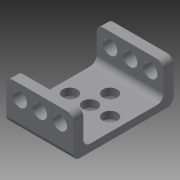
# Autodesk Inventor part: Pantilt
Saved by Autodesk Inventor 2014 (Build 180170000, 170)
## iProperties
Created: 2014-03-07
Part Number: Pantilt
Material: Générique
Document SubType Name: Modeling
Designer: Grégoire
Density: 1 g/cm^3
Appearance: Par défaut
Author: Grégoire
Autodesk Inventor part; units mm, degrees
ref_plane "YZ Plane" through (0, 0, 0) normal (1, 0, 0) x (0, 1, 0)
ref_plane "XZ Plane" through (0, 0, 0) normal (0, 1, 0) x (-1, 0, 0)
ref_plane "XY Plane" through (0, 0, 0) normal (0, 0, 1) x (1, 0, 0)
sketch "Esquisse5" plane through (0, 0, 0) normal (0, 0, 1) x (1, 0, 0)
  line L0 (0, 0) -> (20, 0)
  line L1 (20, 0) -> (20, 30)
  line L2 (20, 30) -> (0, 30)
  line L3 (0, 30) -> (0, 0)
  line L4 (10, 0) -> (10, 30) construction
  circle A0 centre (10, 9) radius 2.15
  circle A1 centre (10, 15) radius 2.15
  circle A2 centre (10, 21) radius 2.15
  line L5 (10, 15) -> (20, 15) construction
  circle A3 centre (16, 15) radius 2.15
  circle A4 centre (4, 15) radius 2.15
  circle A5 centre (10, 15) radius 2.15
  dimension "d61" = 20
  dimension "d62" = 30
  dimension "d64" = 4.3
  dimension "d67" = 6
  dimension "d74" = 6
  dimension "d77" = 6
  constraints: 12 end point, 6 centre point, 4 midpoint, 3 horizontal, 2 parallel, 2 perpendicular, 1 coincident, 1 point on line, 1 vertical, 10 other
  measures "d61" distance of L0.start L0.end
  measures "d62" distance of L2.end L0.start
  measures "d64" diameter of A0
  measures "d67" distance of A0.centre L5.start
  measures "d74" distance of L5.start A3.centre
  measures "d77" distance of L5.start A4.centre
extrude "Extrusion5" add sketch "Esquisse5" along normal blind 2.2
sketch "Esquisse9" plane through (0, 0, 2.2) normal (0, 0, 1) x (1, 0, 0)
  line L0 (20, 0) -> (20, 30) construction
  line L1 (0, 30) -> (0, 0) construction
  line L2 (0, 30) -> (20, 30)
  line L3 (20, 30) -> (20, 27)
  line L4 (20, 27) -> (0, 27)
  line L5 (0, 27) -> (0, 30)
  line L6 (0, 15) -> (20, 15) construction
  line L7 (20, 0) -> (0, 0) construction
  line L8 (0, 0) -> (20, 0)
  line L9 (20, 0) -> (20, 3)
  line L10 (20, 3) -> (0, 3)
  line L11 (0, 3) -> (0, 0)
  dimension "d102" = 3
  constraints: 20 end point, 4 symmetric about line, 2 midpoint, 2 parallel, 1 horizontal, 1 perpendicular, 1 point on line
  measures "d102" distance between parallel lines of L2 L4
extrude "Extrusion9" add sketch "Esquisse9" along normal blind 10
sketch "Esquisse10" plane through (0, 0, 0) normal (0, -1, 0) x (1, 0, 0)
  line L0 (0, 0) -> (20, 0) construction
  line L1 (20, 0) -> (20, 12.2) construction
  line L2 (0, 12.2) -> (20, 12.2) construction
  line L3 (10, 12.2) -> (10, 0) construction
  circle A0 centre (10, 8.2) radius 2.15
  line L4 (10, 8.2) -> (20, 8.2) construction
  circle A1 centre (16, 8.2) radius 2.15
  circle A2 centre (4, 8.2) radius 2.15
  circle A3 centre (10, 8.2) radius 2.15
  dimension "d105" = 4
  dimension "d106" = 4.3
  dimension "d109" = 6
  dimension "d112" = 6
  constraints: 4 centre point, 4 end point, 2 horizontal, 2 midpoint, 2 point on line, 1 perpendicular, 6 other
  measures "d105" distance from line of L2 L4.start
  measures "d106" diameter of A0
  measures "d109" distance of L4.start A1.centre
  measures "d112" distance of L4.start A2.centre
extrude "Extrusion10" cut sketch "Esquisse10" against normal through all
fillet "Congé6" radius 2 8 edges at (10, 0, 0) (10, 3, 2.2) (10, 27, 2.2) (0, 28.5, 12.2) (20, 28.5, 12.2) (20, 1.5, 12.2) (0, 1.5, 12.2) (10, 30, 0)
equation "\"d64\" = Holes"
equation "\"d80\" = Depth"
equation "\"d106\" = Holes"
equation "\"Depth\" = 2.2"
equation "\"Holes\" = 4.3"
equation "\"Height\" = 0"
equation "\"Rounding\" = 7"
